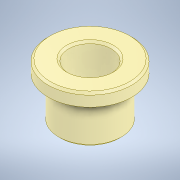
# Autodesk Inventor part: Bøsning_beam_bund
Saved by Autodesk Inventor 2022 (Build 260153000, 153)
## iProperties
Created: 2022-05-04
Part Number: Bøsning_beam_bund
Material: LCP Plastic
Document SubType Name: Modeling
Designer: Patrick
Mass: 2.64995 g
Surface Area: 14.9929 cm^2
Volume: 1.62974 cm^3
Density: 1.626 g/cm^3
Appearance: Nylon 6
Author: Patrick
Autodesk Inventor part; units mm, degrees
ref_plane "YZ Plane" through (0, 0, 0) normal (1, 0, 0) x (0, 1, 0)
ref_plane "XZ Plane" through (0, 0, 0) normal (0, 1, 0) x (-1, 0, 0)
ref_plane "XY Plane" through (0, 0, 0) normal (0, 0, 1) x (1, 0, 0)
sketch "Sketch1" plane through (0, 0, 0) normal (0, 1, 0) x (-1, 0, 0)
  circle A0 centre (0, 0) radius 7.5
  circle A1 centre (0, 0) radius 5.1
  dimension "d0" = 15
  dimension "d1" = 10.2
  constraints: 2 centre point, 2 coincident
  measures "d0" diameter of A0
  measures "d1" diameter of A1
extrude "Extrusion1" add sketch "Sketch1" along normal blind 10
sketch "Sketch2" plane through (0, 10, 0) normal (0, 1, 0) x (1, 0, 0)
  circle A0 centre (0, 0) radius 7.5 projected
  circle A1 centre (0, 0) radius 7.5 projected
  circle A2 centre (0, 0) radius 5.1 projected
  circle A3 centre (0, 0) radius 10
  dimension "d4" = 20
  constraints: 1 centre point, 1 coincident
  measures "d4" diameter of A3
extrude "Extrusion2" add sketch "Sketch2" along normal blind 3 contours A0 | A3
chamfer "Chamfer1" distance 0.5 angle 45 3 edges at (-5.1, 13, 0) (-10, 13, 0) (7.5, 0, 0)
body "Solid1"
